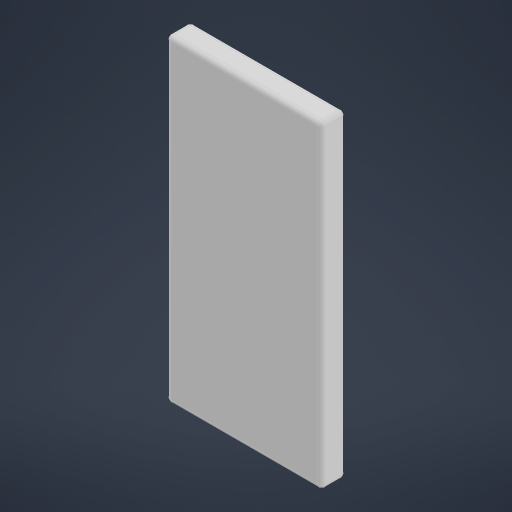
# Autodesk Inventor part: Langbektang houder
Saved by Autodesk Inventor 2023.2 (Build 272271000, 271)
## iProperties
Created: 2020-09-09
Part Number: Langbektang houder
Material: Generic
Document SubType Name: Modeling
Designer: nathan.bollaert
Density: 1 g/cm^3
Appearance: Default
Author: nathan.bollaert
Autodesk Inventor part; units mm, degrees
ref_plane "YZ Plane" through (0, 0, 0) normal (1, 0, 0) x (0, 1, 0)
ref_plane "XZ Plane" through (0, 0, 0) normal (0, 1, 0) x (-1, 0, 0)
ref_plane "XY Plane" through (0, 0, 0) normal (0, 0, 1) x (1, 0, 0)
sketch "Sketch1" plane through (0, 0, 0) normal (0, 0, 1) x (1, 0, 0)
  line L0 (0, -160) -> (78, -160)
  line L1 (78, -160) -> (78, 0)
  line L2 (78, 0) -> (0, 0)
  line L3 (0, 0) -> (0, -160)
  dimension "d228" = 78
  dimension "d229" = 160
  constraints: 8 end point, 2 parallel, 1 coincident, 1 horizontal, 1 perpendicular
  measures "d228" distance of L2.end L1.end
  measures "d229" distance of L1.end L0.end
extrude "Extrusion1" add sketch "Sketch1" along normal blind 12
fillet "Fillet1" radius 2 12 edges at (78, 0, 6) (0, 0, 6) (39, 0, 12) (39, 0, 0) (78, -80, 12) (78, -80, 0) (0, -80, 12) (0, -80, 0) (0, -160, 6) (39, -160, 12) (78, -160, 6) (39, -160, 0)
body "Solid5"
